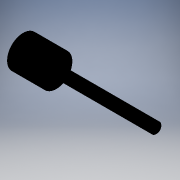
# Autodesk Inventor part: C-0410000_rod
Saved by Autodesk Inventor 2017.3 (Build 213256000, 256)
## iProperties
Part Number: C-0410000_rod
Material: Generic
Catalog Web Link: www.cadenas.de
Description: Standard Air Cylinder_rod-Original Line - Standard Air Cylinders
Vendor: BIMBA
Document SubType Name: Modeling
Designer: partserver
Manufacturer: BIMBA
Mass: 7.69637 g
Surface Area: 29.9125 cm^2
Volume: 7.69637 cm^3
Density: 1 g/cm^3
Appearance: PSOLRGB-0-0-0
Category: PARTsolutions
Company: BIMBA
Title: C-0410000_rod
Author: Cadenas PARTsolutions
Comments: Original Line - Standard Air Cylinders
PSOL_IDENT_0: {$CADENAS_DATA\23d-libs\bimba\bimba_brand\bimba_imperial\bimba_full_line\original_line_cylinders\sta
PSOL_IDENT_1: ndard_air_cylinders\rod.prj},327 {VTYP=3D},{NB=C-0410000_rod},{LINA=C-0410000_rod},{NN=Standard Air
PSOL_IDENT_2: Cylinder_rod},{DATE=19.01.2022 10:19:37},{GEOMDATE=27.08.2019 11:00:52},{VERSION=},{LINEID=50},{WBVA
PSOL_IDENT_3: R=STROKE,ACTING,MNT,DER,NR,BM,CO,M,EE,EEL,K,Q,Y,F,G,T,B,H,SER,SR,NT,W,E,HL,ST,STP,PRC,PB,COLOR1,FCD,
PSOL_IDENT_4: RCD,BCD,ZHJ},{WBNUMERIC=STROKE,EEL,COLOR1,FCD,RCD,BCD,ZHJ}  {NB=C-0410000_rod},{LINA=C-0410000_rod},
PSOL_IDENT_5: {KT=DUMMY},{PN=C-041000},{DASH=},{BORE=0.75000000},{BOREPN=04},{STROKE=1.000},{STROKEALG=[0.001:50/0
PSOL_IDENT_6: .001]},{STROKE1=1.000},{ACTING=},{ACTINGALG= '' , 'Single Acting' , 'R' , 'Reverse Single Acting' , '
PSOL_IDENT_7: D' , 'Double Acting' },{ACTINGPN=},{MNT=},{MNTALG= '' , 'Front Nose Mounting' , 'P' , 'Rear Pivot Mo
PSOL_IDENT_8: unting' , 'BF' , 'Front Block Mounting' , 'BR' , 'Rear Block Mounting for Vertical Positioning' , 'B
PSOL_IDENT_9: FT' , 'Front Block Trunnion Mounting' , 'BRT' , 'Rear Block Trunnion Mounting' , 'A' , 'Double End M
PSOL_IDENT_10: ounting with Brackets and Adjustable Stroke' , 'AP' , 'Rear Pivot Mounting with Adjustable Stroke' }
PSOL_IDENT_11: ,{TYPE=C-},{MNTPN=},{DER=},{DERALG= '' , 'N/A' },{NR=},{NRALG= '' , 'Standard' , 'NR' , 'Non-rotatin
PSOL_IDENT_12: g - Hexagon Rod' },{NRPN=},{BM=},{BMALG= '' , 'Without Built-in Midget 3-Way Solenoid Operated Valve'
PSOL_IDENT_13: , 'LS' , 'With Built-in Midget 3-Way Solenoid Operated Valve' },{BMPN=},{CO=},{COALG= '' , 'N/A' },
PSOL_IDENT_14: {M=},{MALG= '', 'Without Magnet', 'M', 'With Magnet' },{EE=},{EEL=0},{EEMAX=11},{EEALG= '', 'Without
PSOL_IDENT_15: Extra Extension', 'EE', 'With Extra Extension' },{EELALG=0},{EEPN=},{EEPN1=0.000},{K=},{KALG= '' , '
PSOL_IDENT_16: N/A' },{KPN=},{Q=},{QALG= '' , 'Without Side Ported Rear Head' , 'Q' , 'With Side Ported Rear Head'
PSOL_IDENT_17: },{QPN=},{Y=},{YALG= '' , 'N/A' },{YPN=},{F=},{FALG= '', 'Standard', 'F', 'Molycoated Body' },{FPN=}
PSOL_IDENT_18: ,{G=},{GPN=},{T=},{TALG= '' , 'Standard' , 'N' , 'Low Temperature' , 'V' , 'High Temperature' },{NPN=
PSOL_IDENT_19: },{VPN=},{B=},{BALG= '', 'Without Bumper' , 'B' , 'With Bumper' },{BPN=},{H=},{HALG= '', 'Standard',
PSOL_IDENT_20: 'H', 'With Heavy Springs' },{HPN=},{SER=},{SERALG= '' , 'N/A' },{SR=C},{SRALG= 'C' , 'Carbon Steel
PSOL_IDENT_21: Rod' , 'SR' , '303 Stainless Steel Rod' , '' , '303 Stainless Steel Rod1' },{SRPN=C},{SRCON=1},{NT=}
PSOL_IDENT_22: ,{NTPN=},{W=},{WALG= '' , 'N/A' },{WPN=},{E=},{EALG= '' , 'Without Special Lube and Seals' , 'E' , '
PSOL_IDENT_23: With Special Lube and Seals' },{EPN=},{HL=},{HLALG= '' , 'N/A' },{ST=},{STALG= '' , 'Without Switch
PSOL_IDENT_24: Track' , 'T' , 'With Switch Track' },{STP=},{STPALG= '' , 'N/A' },{STPN=},{PRC=},{PRCALG= '' , 'With
PSOL_IDENT_25: out Piston Rod Clevis' , 'D-166-1' , 'With Piston Rod Clevis' },{PRCPN=},{PB=},{PBALG= '' , 'Without
PSOL_IDENT_26: Pivot Bracket' , 'D-167' , 'With Pivot Bracket' },{PBPN=},{TLEN=2.2560},{TEXT=0.166667},{SPACE=0.09
PSOL_IDENT_27: 5238},{FRAC=3.8800},{RGCON=},{RGDACCON=},{RHCON=},{RHCONON=1},{RHACCON=},{FNUTCON=1},{RNUTCON=0},{FN
PSOL_IDENT_28: UTPN=D-98},{RNUTPN=},{FNUTTRANS=0.0000},{RNUTTRANS=0.0000},{VHOLECON=2},{A1=0.8750},{A1N=0.8750},{A1
PSOL_IDENT_29: P=1.5940},{A1B=1.5940},{A4=0.3130},{A4N=0.3130},{A4P=0.2525},{A5=0.0300},{A1H=0.531},{A1NH=0.5310},{
PSOL_IDENT_30: A1PH=1.5940},{A1BH=1.0940},{A1SH=1.2190},{A2H=0.2190},{A2NH=0.2190},{LENGTH=1.5000},{LENGTH1=1.5000}
PSOL_IDENT_31: ,{LENGTH2=3.0300},{MUL=1.6900},{MUL11=1.6900},{MUL22=2.6900},{MUL33=1.6900},{MUL2=1.6900},{MUL211=1.
PSOL_IDENT_32: 6900},{MUL222=2.6900},{MUL233=1.6900},{SSS=2.0000},{RGLEN=0.5920},{RHLEN=0.3420},{SSS1=2.0000},{A13=
PSOL_IDENT_33: 1.3120},{THDLEN1=0.5000},{THD1=0.2500},{TAB=UNF},{THDLEN=0.5000},{THD=0.2500},{OD=0.7615},{RODL=3.15
PSOL_IDENT_34: 90},{PL=0.7840},{RODDIA=0.2500},{HEX=0.2500},{RODTRANS=0.0000},{G1=0.1250},{ON=0},{G5=0.6250},{DERLE
PSOL_IDENT_35: N=2.3750},{THOLE=0.0000},{WF=0.2200},{BADD=0.0000},{MADD=0.0000},{NVADD=0.000},{JRADD=0.00000},{COLO
PSOL_IDENT_36: R=0.00,0.00,0.00,0.00},{GROOVE=1},{HOL=0},{D7=0.2520},{H1=1.1175},{D1=0.8050},{D1RH=0.8050},{D1P=0.8
PSOL_IDENT_37: 325},{D1B=0.8625},{D1N=0.8050},{D1NRH=0.8050},{D1BRH=0.8325},{D1PRH=0.8625},{BOZO=0},{HADD=0.000},{C
PSOL_IDENT_38: OLOR1=0},{DEFL=0.0000},{HEXL=0.0000},{SSADD=0.0000},{WFL=0.0000},{MOVE=0.0000},{PRCL2=0.50000},{PRCB=
PSOL_IDENT_39: 0.16000},{PRCTRANS=0.16000},{FCD=0},{RCD=0},{BCD=0},{ZHJ=0.000}
NB: C-0410000_rod
NN: Standard Air Cylinder_rod
NT: Standard
NBSYN: $PN.$COLOR1._rod
LINA: C-0410000_rod
CATALOG: Bimba Products
PN: C-041000
BORE: 0.75
BOREPN: 04
STROKE: 1
ACTING: Single Acting
MNT: Front Nose Mounting
DER: N/A
NR: Standard
BM: Without Built-in Midget 3-Way Solenoid Operated Valve
CO: N/A
M: Without Magnet
EE: Without Extra Extension
EEL: 0
K: N/A
Q: Without Side Ported Rear Head
Y: N/A
F: Standard
G: Without Magnalube Lubrication
T: Standard
B: Without Bumper
H: Standard
SER: N/A
SR: Carbon Steel Rod
W: N/A
E: Without Special Lube and Seals
HL: N/A
ST: Without Switch Track
STP: N/A
PRC: Without Piston Rod Clevis
PB: Without Pivot Bracket
A1N: 0.875
A1P: 1.594
A1B: 1.594
A4N: 0.313
A4P: 0.2525
A5: 0.03
A1NH: 0.531
A1PH: 1.594
A1BH: 1.094
A1SH: 1.219
A2NH: 0.219
A13: 1.312
THDLEN1: 0.5
THD1: 0.25
TAB: UNF
OD: 0.7615
RODDIA: 0.25
HEX: 0.25
G1: 0.125
G5: 0.625
THOLE: 0
WF: 0.22
GROOVE: 1
D7: 0.252
D1P: 0.8325
D1B: 0.8625
D1N: 0.805
D1NRH: 0.805
D1BRH: 0.8325
D1PRH: 0.8625
COLOR1: 0
FCD: 0
RCD: 0
BCD: 0
ZHJ: 0
SUPPLIER: BIMBA
ARTICLENO: C-0410000_rod
BOMINFO: C-0410000_rod
CREATOR: CADENAS GmbH
Autodesk Inventor part; units mm, degrees
ref_plane "YZ Plane" through (0, 0, 0) normal (1, 0, 0) x (0, 1, 0)
ref_plane "XZ Plane" through (0, 0, 0) normal (0, 1, 0) x (-1, 0, 0)
ref_plane "XY Plane" through (0, 0, 0) normal (0, 0, 1) x (1, 0, 0)
sketch "Sketch_1" plane through (0, 0, 0) normal (0, 0, 1) x (1, 0, 0)
  line L0 (67.5386, 0) -> (0, 0)
  line L1 (0, 0) -> (0, 3.175)
  line L2 (0, 3.175) -> (47.625, 3.175)
  line L3 (47.625, 3.175) -> (47.625, 9.6202)
  line L4 (47.625, 9.6202) -> (67.5386, 9.6202)
  line L5 (67.5386, 9.6202) -> (67.5386, 0)
  line L6 (67.5386, 0) -> (0, 0)
  constraints: 14 end point
revolve "Revolution1" add sketch "Sketch_1" angle 360 about axis through (67.5386, 0, 0) along (1, 0, 0)
sketch "Sketch_3" plane through (0, 0, 0) normal (0, 0, 1) x (1, 0, 0)
  line L0 (0, 0) -> (-12.7, 0)
  line L1 (-12.7, 0) -> (-12.7, 2.634)
  line L2 (-12.7, 2.634) -> (-12.159, 3.175)
  line L3 (-12.159, 3.175) -> (0, 3.175)
  line L4 (0, 3.175) -> (0, 0)
  line L5 (0, 0) -> (-12.7, 0)
  constraints: 12 end point
revolve "Revolution2" add sketch "Sketch_3" angle 360 about axis through (0, 0, 0) along (1, 0, 0)
sketch "Sketch_30" plane through (0, 0, 0) normal (0, 0, 1) x (1, 0, 0)
  line L0 (0, 0) -> (-0.254, 0)
  line L1 (-0.254, 2.921) -> (0, 2.921)
  line L2 (0, 2.921) -> (0, 3.429)
  line L3 (0, 3.429) -> (-0.254, 3.429)
  line L4 (-0.254, 3.429) -> (-0.254, 2.921)
  constraints: 10 end point
revolve "Revolution3" cut sketch "Sketch_30" angle 360 about axis through (0, 0, 0) along (1, 0, 0)
ref_plane "dia1_XY" through (0, 3.175, 0) normal (1, 0, 0) x (0, 0, -1)
ref_plane "dia1_YZ" through (0, 3.175, 0) normal (0, 0, -1) x (0, 1, 0)
ref_plane "dia1_ZX" through (0, 3.175, 0) normal (0, 1, 0) x (1, 0, 0)
ref_plane "dia12_XY" through (0, 0, 10.2235) normal (1, 0, 0) x (0, 0, -1)
ref_plane "dia12_YZ" through (0, 0, 10.2235) normal (0, 0, -1) x (0, 1, 0)
ref_plane "dia12_ZX" through (0, 0, 10.2235) normal (0, 1, 0) x (1, 0, 0)
ref_plane "dia2_XY" through (0, -3.175, 0) normal (1, 0, 0) x (0, 0, -1)
ref_plane "dia2_YZ" through (0, -3.175, 0) normal (0, 0, -1) x (0, 1, 0)
ref_plane "dia2_ZX" through (0, -3.175, 0) normal (0, 1, 0) x (1, 0, 0)
ref_plane "dia22_XY" through (0, 0, -10.2235) normal (1, 0, 0) x (0, 0, -1)
ref_plane "dia22_YZ" through (0, 0, -10.2235) normal (0, 0, -1) x (0, 1, 0)
ref_plane "dia22_ZX" through (0, 0, -10.2235) normal (0, 1, 0) x (1, 0, 0)
ref_plane "rl1_XY" through (-12.7, 0, 0) normal (1, 0, 0) x (0, 0, -1)
ref_plane "rl1_YZ" through (-12.7, 0, 0) normal (0, 0, -1) x (0, 1, 0)
ref_plane "rl1_ZX" through (-12.7, 0, 0) normal (0, 1, 0) x (1, 0, 0)
ref_plane "rl2_XY" through (0, 0, 0) normal (1, 0, 0) x (0, 0, -1)
ref_plane "rl2_YZ" through (0, 0, 0) normal (0, 0, -1) x (0, 1, 0)
ref_plane "rl2_ZX" through (0, 0, 0) normal (0, 1, 0) x (1, 0, 0)
ref_plane "rod_cp_XY" through (0, 0, 0) normal (1, 0, 0) x (0, 0, -1)
ref_plane "rod_cp_YZ" through (0, 0, 0) normal (0, 0, -1) x (0, 1, 0)
ref_plane "rod_cp_ZX" through (0, 0, 0) normal (0, 1, 0) x (1, 0, 0)
ref_plane "thd1_XY" through (-12.7, 3.175, 0) normal (1, 0, 0) x (0, 0, -1)
ref_plane "thd1_YZ" through (-12.7, 3.175, 0) normal (0, 0, -1) x (0, 1, 0)
ref_plane "thd1_ZX" through (-12.7, 3.175, 0) normal (0, 1, 0) x (1, 0, 0)
ref_plane "thd2_XY" through (-12.7, -3.175, 0) normal (1, 0, 0) x (0, 0, -1)
ref_plane "thd2_YZ" through (-12.7, -3.175, 0) normal (0, 0, -1) x (0, 1, 0)
ref_plane "thd2_ZX" through (-12.7, -3.175, 0) normal (0, 1, 0) x (1, 0, 0)
ref_plane "to_rod_clevis_XY" through (-16.764, 0, 0) normal (1, 0, 0) x (0, 0, -1)
ref_plane "to_rod_clevis_YZ" through (-16.764, 0, 0) normal (0, 0, -1) x (0, 1, 0)
ref_plane "to_rod_clevis_ZX" through (-16.764, 0, 0) normal (0, 1, 0) x (1, 0, 0)
body "Solid1"
